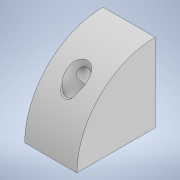
# Autodesk Inventor part: 鋁擠固定器小
Saved by Autodesk Inventor 2021 (Build 250183000, 183)
## iProperties
Created: 2023-03-06
Part Number: 鋁擠固定器小
Material: 一般
Document SubType Name: Modeling
Designer: brian
Density: 1 g/cm^3
Appearance: 預設
Author: brian
Autodesk Inventor part; units mm, degrees
ref_plane "YZ Plane" through (0, 0, 0) normal (1, 0, 0) x (0, 1, 0)
sketch "草圖1" plane through (0, 0, 0) normal (1, 0, 0) x (0, 1, 0)
  line L0 (0, 0) -> (0, 30)
  arc A0 (30, 0) -> (0, 30) centre (0, 0) ccw
  line L1 (30, 0) -> (0, 0)
  dimension "d0" = 30
  constraints: 4 end point, 2 line through centre, 2 point on circle, 1 centre point, 1 perpendicular, 1 point on line, 1 vertical
  measures "d0" radius of A0
extrude "擠出1" add sketch "草圖1" along normal blind 20
ref_plane "工作平面1" through (0, 30, 0) normal (0, -1, 0) x (1, 0, 0)
sketch "草圖2" plane through (0, 30, 0) normal (0, -1, 0) x (1, 0, 0)
  line L0 (0, 0) -> (20, 0) projected
  point P0 (10, 20)
  point P1 (10, 0)
  dimension "d3" = 20
  constraints: 1 midpoint, 1 vertical alignment
  measures "d3" distance from line of L0 point (10, 20)
hole "孔1" at (10, 30, 20) direction (0, -1, 0) diameter 4 end through all counterbore diameter 8 counterbore depth 25
ref_plane "工作平面2" through (10, 0, 30) normal (0, 0, -1) x (-1, 0, 0)
sketch "草圖3" plane through (10, 0, 30) normal (0, 0, -1) x (-1, 0, 0)
  line L0 (10, 0) -> (-10, 0) projected
  point P0 (0, 20)
  point P1 (0, 0)
  dimension "d11" = 20
  constraints: 1 midpoint, 1 vertical alignment
  measures "d11" distance from line of L0 point (0, 20)
hole "孔2" at (10, 20, 30) direction (0, 0, -1) diameter 3 end through all counterbore diameter 6 counterbore depth 25
